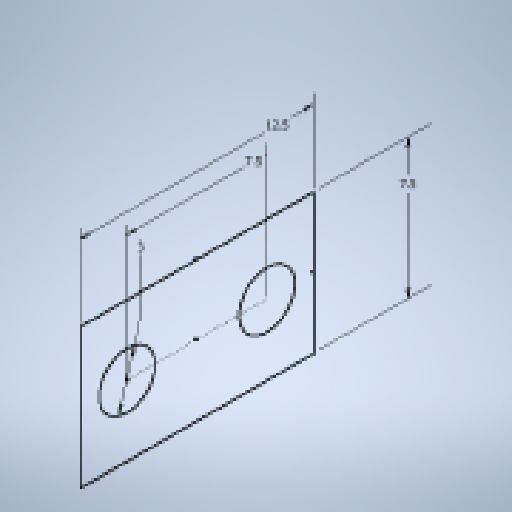
# Autodesk Inventor part: LJ12_Adapter
Saved by Autodesk Inventor 2023 (Build 270158000, 158)
## iProperties
Created: 2022-05-30
Part Number: LJ12_Adapter
Material: Generic
Document SubType Name: Modeling
Designer: plebbb
Density: 1 g/cm^3
Appearance: Default
Author: plebbb
Autodesk Inventor part; units mm, degrees
ref_plane "YZ Plane" through (0, 0, 0) normal (1, 0, 0) x (0, 1, 0)
ref_plane "XZ Plane" through (0, 0, 0) normal (0, 1, 0) x (-1, 0, 0)
ref_plane "XY Plane" through (0, 0, 0) normal (0, 0, 1) x (1, 0, 0)
sketch "Sketch1" plane through (0, 0, 0) normal (1, 0, 0) x (0, 1, 0)
  line L0 (0, 0) -> (7.5, 0)
  line L1 (7.5, 0) -> (7.5, -12.5)
  line L2 (7.5, -12.5) -> (0, -12.5)
  line L3 (0, -12.5) -> (0, 0)
  circle A0 centre (2.5, -2.5) radius 1.5
  circle A1 centre (2.5, -10) radius 1.5
  line L4 (2.5, -2.5) -> (2.5, -10) construction
  line L5 (7.5, -12.5) -> (7.5, 0)
  point P0 (2.5, -6.25)
  point P1 (7.5, -6.25)
  point P2 (3.75, -12.5)
  dimension "d0" = 12.5
  dimension "d1" = 7.5
  dimension "d2" = 3
  dimension "d3" = 7.5
  dimension "d4" = 5
  constraints: 12 end point, 3 midpoint, 2 centre point, 2 parallel, 1 coincident, 1 equal radius, 1 horizontal, 1 horizontal alignment, 1 perpendicular, 1 vertical
  measures "d0" distance of L0.end L1.end
  measures "d1" distance of L1.end L2.end
  measures "d2" diameter of A0
  measures "d3" distance of L4.start L4.end
  measures "d4" distance from line of point (7.5, -6.25) L4
extrude "Extrusion1" add sketch "Sketch1" along normal blind 5
sketch "Sketch2" plane through (5, 0, 0) normal (1, 0, 0) x (0, 0, -1)
  line L0 (12.5, 7.5) -> (0, 7.5) projected
  line L1 (0, 7.5) -> (0, 0) projected
  line L2 (0, 7.5) -> (0, 52.5)
  line L3 (0, 52.5) -> (10, 52.5)
  line L4 (10, 52.5) -> (10, 7.5)
  dimension "d7" = 10
  dimension "d8" = 45
  constraints: 6 end point, 2 perpendicular, 1 point on line, 1 vertical
  measures "d7" distance of L2.end L3.end
  measures "d8" distance of L3.end L4.end
extrude "Extrusion2" add sketch "Sketch2" against normal blind 5
sketch "Sketch3" plane through (5, 7.5, -10) normal (0, 0, -1) x (-1, 0, 0)
  circle A0 centre (5, 53.6603) radius 10
  circle A1 centre (5, 53.6603) radius 6
  line L0 (0, 45) -> (5, 45) projected
  point P0 (5, -7.5)
  point P1 (2.5, 45)
  dimension "d11" = 12
  dimension "d12" = 4
  constraints: 1 centre point, 1 coincident, 1 midpoint, 1 vertical alignment, 3 other
  measures "d11" diameter of A1
extrude "Extrusion3" add sketch "Sketch3" against normal up to surface (10 mm away)
fillet "Fillet1" radius 5 3 edges at (5, 52.5, -5) (0, 51.1603, -5) (2.5, 7.5, -10)
body "Solid1"
